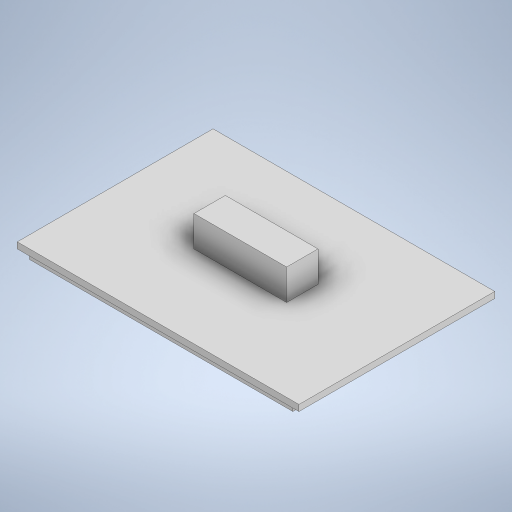
# Autodesk Inventor part: Lid
Saved by Autodesk Inventor 2024 (Build 280153000, 153)
## iProperties
Created: 2025-02-03
Part Number: Lid
Material: Generic
Document SubType Name: Modeling
Designer: matsk
Density: 1 g/cm^3
Appearance: Default
Author: matsk
Autodesk Inventor part; units mm, degrees
ref_plane "YZ Plane" through (0, 0, 0) normal (1, 0, 0) x (0, 1, 0)
ref_plane "XZ Plane" through (0, 0, 0) normal (0, 1, 0) x (-1, 0, 0)
ref_plane "XY Plane" through (0, 0, 0) normal (0, 0, 1) x (1, 0, 0)
sketch "Sketch1" plane through (0, 0, 0) normal (0, 1, 0) x (-1, 0, 0)
  line L0 (0, 0) -> (-42.9, 0)
  line L1 (-42.9, 0) -> (-42.9, -29.75)
  line L2 (-42.9, -29.75) -> (0, -29.75)
  line L3 (0, -29.75) -> (0, 0)
  dimension "d0" = 42.9
  dimension "d1" = 29.75
  constraints: 8 end point, 2 parallel, 1 horizontal, 1 perpendicular
  measures "d0" distance of L2.end L1.end
  measures "d1" distance of L1.end L0.end
extrude "Extrusion1" add sketch "Sketch1" along normal blind 1
sketch "Sketch2" plane through (0, 1, 0) normal (0, 1, 0) x (1, 0, 0)
  line L0 (42.9, 0) -> (42.9, 29.75) projected
  line L1 (42.9, 29.75) -> (0, 29.75) projected
  line L2 (-1.5, 31.392) -> (44.4, 31.392)
  line L3 (44.4, 31.392) -> (44.4, -0.507)
  line L4 (44.4, -0.507) -> (-1.5, -0.507)
  line L5 (-1.5, -0.507) -> (-1.5, 31.392)
  point P0 (0, 0)
  constraints: 8 end point, 2 parallel, 1 horizontal, 1 perpendicular
extrude "Extrusion2" add sketch "Sketch2" along normal blind 1
sketch "Sketch3" plane through (0, 2, 0) normal (0, 1, 0) x (1, 0, 0)
  line L0 (-1.5, -0.507) -> (44.4, -0.507) projected
  line L1 (44.4, 31.392) -> (-1.5, 31.392) projected
  line L2 (-1.5, -0.507) -> (44.4, 31.392)
  line L3 (44.4, -0.507) -> (44.4, 31.392) projected
  line L4 (44.4, -0.507) -> (-1.5, 31.392)
  line L5 (13.9, 12.885) -> (29, 12.885)
  line L6 (29, 12.885) -> (29, 18)
  line L7 (29, 18) -> (13.9, 18)
  line L8 (13.9, 18) -> (13.9, 12.885)
  line L9 (13.9, 12.885) -> (29, 18) construction
  line L10 (29, 12.885) -> (13.9, 18) construction
  point P0 (0, 0)
  point P1 (21.45, 15.4425)
  constraints: 16 end point, 3 midpoint, 2 parallel, 1 horizontal, 1 perpendicular
extrude "Extrusion3" add sketch "Sketch3" along normal blind 5 contours L5 L8 L7 L4 L2 | L2 L4 L5 | L4 L2 L7 L6 L5 | L4 L7 L2
body "Solid1"
